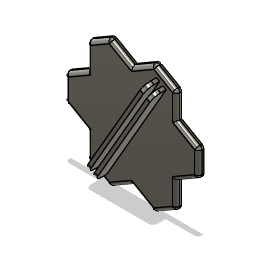
Hex Base Huge (Autodesk Fusion 360 design; units mm, degrees)
Autodesk Fusion 360 part; units mm, degrees
sketch "Sketch3" plane through (0, 0, 0) normal (0, 0, 1) x (1, 0, 0)
  line L0 (12.2, 7.0437) -> (0, 14.0873)
  line L1 (0, 14.0873) -> (-12.2, 7.0437)
  line L2 (-12.2, 7.0437) -> (-12.2, -7.0437)
  line L3 (-12.2, -7.0437) -> (0, -14.0873)
  line L4 (0, -14.0873) -> (12.2, -7.0437)
  line L5 (12.2, -7.0437) -> (12.2, 7.0437)
  line L6 (0, -14.0873) -> (0, 14.0873) construction
  line L7 (24.4, 14.0873) -> (24.4, 28.1747)
  line L8 (24.4, 28.1747) -> (12.2, 35.2184)
  line L9 (12.2, 35.2184) -> (0, 28.1747)
  line L10 (0, 28.1747) -> (0, 14.0873)
  line L11 (0, 14.0873) -> (12.2, 7.0437)
  line L12 (12.2, 7.0437) -> (24.4, 14.0873)
  line L13 (0, 14.0873) -> (0, 28.1747)
  line L14 (0, 28.1747) -> (-12.2, 35.2184)
  line L15 (-12.2, 35.2184) -> (-24.4, 28.1747)
  line L16 (-24.4, 28.1747) -> (-24.4, 14.0873)
  line L17 (-24.4, 14.0873) -> (-12.2, 7.0437)
  line L18 (-12.2, 7.0437) -> (0, 14.0873)
  line L19 (36.6, -7.0437) -> (36.6, 7.0437)
  line L20 (36.6, 7.0437) -> (24.4, 14.0873)
  line L21 (24.4, 14.0873) -> (12.2, 7.0437)
  line L22 (12.2, 7.0437) -> (12.2, -7.0437)
  line L23 (12.2, -7.0437) -> (24.4, -14.0873)
  line L24 (24.4, -14.0873) -> (36.6, -7.0437)
  line L25 (-12.2, 7.0437) -> (-24.4, 14.0873)
  line L26 (-24.4, 14.0873) -> (-36.6, 7.0437)
  line L27 (-36.6, 7.0437) -> (-36.6, -7.0437)
  line L28 (-36.6, -7.0437) -> (-24.4, -14.0873)
  line L29 (-24.4, -14.0873) -> (-12.2, -7.0437)
  line L30 (-12.2, -7.0437) -> (-12.2, 7.0437)
  line L31 (-12.2, -7.0437) -> (-24.4, -14.0873)
  line L32 (-24.4, -14.0873) -> (-24.4, -28.1747)
  line L33 (-24.4, -28.1747) -> (-12.2, -35.2184)
  line L34 (-12.2, -35.2184) -> (0, -28.1747)
  line L35 (0, -28.1747) -> (0, -14.0873)
  line L36 (0, -14.0873) -> (-12.2, -7.0437)
  line L37 (24.4, -14.0873) -> (12.2, -7.0437)
  line L38 (12.2, -7.0437) -> (0, -14.0873)
  line L39 (0, -14.0873) -> (0, -28.1747)
  line L40 (0, -28.1747) -> (12.2, -35.2184)
  line L41 (12.2, -35.2184) -> (24.4, -28.1747)
  line L42 (24.4, -28.1747) -> (24.4, -14.0873)
  line L43 (0, 48) -> (0, -40) construction
  point P0 (12.2, 21.131)
  point P1 (-12.2, 21.131)
  point P2 (24.4, 0)
  point P3 (-24.4, 0)
  point P4 (-12.2, -21.131)
  point P5 (12.2, -21.131)
  dimension "d10" = 12.2
  dimension "d29" = 12.2
  dimension "d30" = 12.2
  dimension "d31" = 12.2
  dimension "d32" = 12.2
  dimension "d33" = 12.2
  dimension "d34" = 12.2
  constraint vertical L6
  constraint collinear L1 L18
  constraint collinear L0 L11
  constraint collinear L10 L13
  constraint collinear L5 L22
  constraint collinear L12 L21
  constraint collinear L23 L37
  constraint collinear L4 L38
  constraint collinear L35 L39
  constraint collinear L3 L36
  constraint collinear L29 L31
  constraint collinear L2 L30
  constraint parallel L6 L43
  constraint collinear L13 L43
  constraint coincident origin L43
  measures "d10" distance of origin L5
  measures "d29" distance of P0 L12
  measures "d30" distance of P1 L18
  measures "d31" distance of P2 L24
  measures "d32" distance of P3 L30
  measures "d33" distance of P4 L36
  measures "d34" distance of P5 L42
extrude "Extrude2" add sketch "Sketch3" along normal blind 3
sketch "Sketch4" plane through (0, 0, 3) normal (0, 0, 1) x (1, 0, 0)
  line L0 (13.5653, 29.6958) -> (-18.9347, -26.5958)
  line L1 (-18.9347, -26.5958) -> (-17.2026, -27.5958)
  line L2 (-17.2026, -27.5958) -> (15.2974, 28.6958)
  line L3 (15.2974, 28.6958) -> (13.5653, 29.6958)
  line L4 (17.2026, 27.5958) -> (-15.2974, -28.6958)
  line L5 (-15.2974, -28.6958) -> (-13.5653, -29.6958)
  line L6 (-13.5653, -29.6958) -> (18.9347, 26.5958)
  line L7 (18.9347, 26.5958) -> (17.2026, 27.5958)
  line L8 (-24.4, 14.0873) -> (24.4, -14.0873) construction
  line L9 (24.4, -28.1747) -> (24.4, -14.0873)
  line L10 (24.4, -14.0873) -> (36.6, -7.0437)
  line L11 (36.6, -7.0437) -> (36.6, 7.0437)
  line L12 (36.6, 7.0437) -> (24.4, 14.0873)
  line L13 (24.4, 14.0873) -> (24.4, 28.1747)
  line L14 (24.4, 28.1747) -> (12.2, 35.2184)
  line L15 (12.2, 35.2184) -> (0, 28.1747)
  line L16 (0, 28.1747) -> (-12.2, 35.2184)
  line L17 (-12.2, 35.2184) -> (-24.4, 28.1747)
  line L18 (-24.4, 28.1747) -> (-24.4, 14.0873)
  line L19 (-24.4, 14.0873) -> (-36.6, 7.0437)
  line L20 (-36.6, 7.0437) -> (-36.6, -7.0437)
  line L21 (-36.6, -7.0437) -> (-24.4, -14.0873)
  line L22 (-24.4, -14.0873) -> (-24.4, -28.1747)
  line L23 (-24.4, -28.1747) -> (-12.2, -35.2184)
  line L24 (-12.2, -35.2184) -> (0, -28.1747)
  line L25 (0, -28.1747) -> (12.2, -35.2184)
  line L26 (12.2, -35.2184) -> (24.4, -28.1747)
  line L27 (18.3, 31.6965) -> (-18.3, -31.6965)
  dimension "d13" = 65
  dimension "d14" = 2
  dimension "d15" = 2.2
  constraint perpendicular L0 L1
  constraint parallel L0 L2
  constraint parallel L1 L3
  constraint perpendicular L4 L5
  constraint parallel L4 L6
  constraint parallel L5 L7
  constraint equal L0 L4
  constraint parallel L0 L4
  constraint equal L3 L7
  constraint collinear L3 L7
  constraint coincident origin L8
  constraint symmetric L1 L3 L8
  constraint coincident L8.end L9.end
  constraint coincident L8.start L18.end
  constraint midpoint L14 L27.start
  constraint midpoint L23 L27.end
  constraint symmetric L2 L4 L27
  measures "d13" distance of L0.start L0.end
  measures "d14" distance of L0.start L2.end
  measures "d15" distance of L2 L4
extrude "Extrude3" add sketch "Sketch4" along normal blind 7 contours L0 L1 L2 L3 | L4 L5 L6 L7
sketch "Sketch5" plane through (0, 0, 0) normal (0, 0, -1) x (-1, 0, 0)
  line L0 (-17.2026, 27.5958) -> (-15.2974, 28.6958)
  line L1 (-15.2974, 28.6958) -> (17.2026, -27.5958)
  line L2 (17.2026, -27.5958) -> (15.2974, -28.6958)
  line L3 (15.2974, -28.6958) -> (-17.2026, 27.5958)
  line L4 (24.4, -28.1747) -> (12.2, -35.2184)
  line L5 (-24.4, 28.1747) -> (-12.2, 35.2184)
  line L6 (18.3, -31.6965) -> (-18.3, 31.6965) construction
  line L7 (24.4, 14.0873) -> (-24.4, -14.0873) construction
  line L8 (24.4, 14.0873) -> (36.6, 7.0437)
  point P0 (24.4, 14.0873)
  point P1 (-24.4, -14.0873)
  dimension "d18" = 65
  dimension "d19" = 2.2
  constraint perpendicular L2 L3
  constraint perpendicular L0 L1
  constraint perpendicular L0 L3
  constraint midpoint L4 L6.start
  constraint midpoint L5 L6.end
  constraint coincident P0 L7.start
  constraint coincident P1 L7.end
  constraint symmetric L1 L3 L6
  constraint symmetric L0 L2 L7
  measures "d18" distance of L0.start L2.end
  measures "d19" distance of L0.start L0.end
extrude "Extrude4" cut sketch "Sketch5" against normal blind 2
fillet "Fillet1" radius 4 4 edges at (-14.4313, -29.1958, 10) (-18.0687, -27.0958, 10) (18.0687, 27.0958, 10) (14.4313, 29.1958, 10)
fillet "Fillet2" radius 2 12 edges at (-12.2, -35.2184, 1.5) (12.2, -35.2184, 1.5) (24.4, -28.1747, 1.5) (36.6, -7.0437, 1.5) (36.6, 7.0437, 1.5) (24.4, 28.1747, 1.5) (12.2, 35.2184, 1.5) (-12.2, 35.2184, 1.5) (-24.4, 28.1747, 1.5) (-36.6, 7.0437, 1.5) (-36.6, -7.0437, 1.5) (-24.4, -28.1747, 1.5)
fillet "Fillet3" radius 0.5 4 edges at (-16.25, -28.1458, 0) (-0.9526, 0.55, 0) (16.25, 28.1458, 0) (0.9526, -0.55, 0)
fillet "Fillet5" radius 2 30 edges at (-5.6, 31.4079, 3) (-12.2, 34.909, 3) (-18.3, 31.6965, 3) (-24.1321, 28.02, 3) (-24.4, 20.5537, 3) (24.4, 20.5537, 3) (24.1321, 28.02, 3) (18.3, 31.6965, 3) (12.2, 34.909, 3) (5.6, 31.4079, 3) (30, -10.8542, 3) (36.3321, -6.889, 3) (36.6, 0, 3) (36.3321, 6.889, 3) (30, 10.8542, 3) (5.6, -31.4079, 3) (12.2, -34.909, 3) (18.3, -31.6965, 3) (24.1321, -28.02, 3) (24.4, -20.5537, 3) (-24.4, -20.5537, 3) (-24.1321, -28.02, 3) (-18.3, -31.6965, 3) (-12.2, -34.909, 3) (-5.6, -31.4079, 3) (-30, 10.8542, 3) (-36.3321, 6.889, 3) (-36.6, 0, 3) (-36.3321, -6.889, 3) (-30, -10.8542, 3)
named bodies: "Hex Base Huge"
